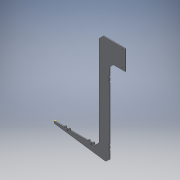
# Autodesk Inventor part: Z stage_side
Saved by Autodesk Inventor 2019 (Build 230136000, 136)
## iProperties
Created: 2020-03-07
Part Number: Z stage_side
Material: Generic
Document SubType Name: Modeling
Designer: Vijay
Density: 1 g/cm^3
Appearance: Default
Author: Vijay
Autodesk Inventor part; units mm, degrees
ref_plane "YZ Plane" through (0, 0, 0) normal (1, 0, 0) x (0, 1, 0)
ref_plane "XZ Plane" through (0, 0, 0) normal (0, 1, 0) x (-1, 0, 0)
ref_plane "XY Plane" through (0, 0, 0) normal (0, 0, 1) x (1, 0, 0)
sketch "Sketch1" plane through (0, 0, 0) normal (0, 0, 1) x (1, 0, 0)
  line L0 (230, 0) -> (0, 0) projected
  line L1 (0, 0) -> (0, -8.9243)
  line L2 (0, -8.9243) -> (282.1829, -48.5825)
  line L3 (282.1829, -48.5825) -> (282.1829, 400)
  line L4 (230, 0) -> (230, 500)
  line L5 (282.1829, 400) -> (362.1829, 400)
  line L6 (230, 500) -> (362.1829, 500)
  line L7 (362.1829, 500) -> (362.1829, 400)
  dimension "d0" = 400
  dimension "d1" = 8
  dimension "d10" = 80
  dimension "d11" = 100
  constraints: 14 end point, 2 horizontal, 2 vertical, 1 parallel, 1 perpendicular
  measures "d0" distance between parallel lines of L0 L5
  measures "d1" angle of L2 L0
  measures "d10" distance between parallel lines of L7 L3
  measures "d11" distance of L6.end L5.end
extrude "Extrusion1" add sketch "Sketch1" along normal blind 4
chamfer "Chamfer1" distance 20 angle 45 2 edges at (230, 500, 2) (282.1829, 400, 2)
chamfer "Chamfer2" distance 20 angle 45 2 edges at (230, 0, 2) (282.1829, -48.5825, 2)
sketch "Sketch2" plane through (0, 0, 0) normal (0, 0, -1) x (-1, 0, 0)
  point P0 (0, 0)
sketch "Sketch3" plane through (0, 0, 0) normal (0, 0, -1) x (-1, 0, 0)
  point P0 (0, 0)
sketch "Sketch4" plane through (0, 0, 0) normal (0, 0, -1) x (-1, 0, 0)
  point P0 (0, 0)
sketch "Sketch5" plane through (0, 0, 0) normal (0, 0, -1) x (-1, 0, 0)
  line L0 (-278.1829, 10.465) -> (-278.1829, 16.465) construction
  line L1 (-282.1829, 16.465) -> (-278.1829, 16.465) construction
  line L2 (-282.1829, 10.465) -> (-282.1829, 16.465) construction
  line L3 (-282.1829, 10.465) -> (-278.1829, 10.465) construction
  line L4 (-278.1829, 31.665) -> (-278.1829, 37.665) construction
  line L5 (-282.1829, 37.665) -> (-278.1829, 37.665) construction
  line L6 (-282.1829, 31.665) -> (-282.1829, 37.665) construction
  line L7 (-282.1829, 31.665) -> (-278.1829, 31.665) construction
  line L8 (-278.1829, 332.8339) -> (-278.1829, 338.8339) construction
  line L9 (-282.1829, 338.8339) -> (-278.1829, 338.8339) construction
  line L10 (-282.1829, 332.8339) -> (-282.1829, 338.8339) construction
  line L11 (-282.1829, 332.8339) -> (-278.1829, 332.8339) construction
  line L12 (-278.1829, 311.6339) -> (-278.1829, 317.6339) construction
  line L13 (-282.1829, 317.6339) -> (-278.1829, 317.6339) construction
  line L14 (-282.1829, 311.6339) -> (-282.1829, 317.6339) construction
  line L15 (-282.1829, 311.6339) -> (-278.1829, 311.6339) construction
  line L16 (-277.9829, 339.0339) -> (-277.9829, 332.6339)
  line L17 (-277.9829, 332.6339) -> (-282.3829, 332.6339)
  line L18 (-282.3829, 332.6339) -> (-282.3829, 339.0339)
  line L19 (-282.3829, 339.0339) -> (-277.9829, 339.0339)
  line L20 (-277.9829, 317.8339) -> (-277.9829, 311.4339)
  line L21 (-277.9829, 311.4339) -> (-282.3829, 311.4339)
  line L22 (-282.3829, 311.4339) -> (-282.3829, 317.8339)
  line L23 (-282.3829, 317.8339) -> (-277.9829, 317.8339)
  line L24 (-277.9829, 37.865) -> (-277.9829, 31.465)
  line L25 (-277.9829, 31.465) -> (-282.3829, 31.465)
  line L26 (-282.3829, 31.465) -> (-282.3829, 37.865)
  line L27 (-282.3829, 37.865) -> (-277.9829, 37.865)
  line L28 (-277.9829, 10.265) -> (-277.9829, 16.665)
  line L29 (-277.9829, 16.665) -> (-282.3829, 16.665)
  line L30 (-282.3829, 16.665) -> (-282.3829, 10.265)
  line L31 (-282.3829, 10.265) -> (-277.9829, 10.265)
  point P0 (0, 0)
  dimension "d24" = 0.2
  dimension "d25" = 0.2
  dimension "d26" = 0.2
  dimension "d27" = 0.2
  constraints: 32 end point, 12 other
  measures "d24" distance between parallel lines of L9 L19
  measures "d25" distance between parallel lines of L13 L23
  measures "d26" distance between parallel lines of L5 L27
  measures "d27" distance between parallel lines of L3 L31
extrude "Extrusion2" cut sketch "Sketch5" against normal blind 25.4
sketch "Sketch6" plane through (0, 0, 0) normal (0, 0, -1) x (-1, 0, 0)
  line L0 (-278.1829, 25.5649) -> (-278.1829, 22.5649) projected
  line L1 (-282.1829, 25.5649) -> (-278.1829, 25.5649) projected
  line L2 (-282.1829, 22.5649) -> (-282.1829, 25.5649) projected
  line L3 (-282.1829, 22.5649) -> (-278.1829, 22.5649) projected
  line L4 (-278.1829, 326.7338) -> (-278.1829, 323.7338) projected
  line L5 (-282.1829, 326.7338) -> (-278.1829, 326.7338) projected
  line L6 (-282.1829, 323.7338) -> (-282.1829, 326.7338) projected
  line L7 (-282.1829, 323.7338) -> (-278.1829, 323.7338) projected
  circle A0 centre (-280.1829, 325.2338) radius 1.6
  circle A1 centre (-280.1829, 24.0649) radius 1.6
  point P0 (0, 0)
  dimension "d14" = 3.2
  dimension "d15" = 3.2
  constraints: 2 centre point
  measures "d14" diameter of A0
  measures "d15" diameter of A1
extrude "Extrusion3" cut sketch "Sketch6" against normal through all contours A1 L3 L1 | L1 A1 | A1 L3 | A0 L7 L5 | L5 A0 | A0 L7
sketch "Sketch7" plane through (0, 0, 0) normal (0, 0, -1) x (-1, 0, 0)
  line L0 (-230, 4.0001) -> (-214.0001, 4.0001) projected
  line L1 (-210, 0) -> (-230, 20) projected
  line L2 (-210, 0) -> (-214.0001, 0)
  line L3 (-214.0001, 0) -> (-214.0001, 4.0001)
  line L4 (-214.0001, 4.0001) -> (-210, 4.0001)
  line L5 (-210, 4.0001) -> (-210, 0)
  point P0 (0, 0)
  constraints: 8 end point, 2 parallel, 2 point on line, 1 horizontal, 1 perpendicular
extrude "Extrusion4" cut sketch "Sketch7" against normal blind 25.4
sketch "Sketch8" plane through (0, 0, 0) normal (0, 0, -1) x (-1, 0, 0)
  line L0 (-209.8759, -14.6536) -> (-209.8759, 0) projected
  line L1 (-168.9242, -14.6536) -> (-209.8759, -14.6536) projected
  line L2 (-168.9242, 0) -> (-168.9242, -14.6536) projected
  line L3 (-175.8001, 0) -> (-168.9242, 0) projected
  line L4 (-175.8001, 6.35) -> (-175.8001, 0) projected
  line L5 (-181.8001, 6.35) -> (-175.8001, 6.35) projected
  line L6 (-181.8001, 0) -> (-181.8001, 6.35) projected
  line L7 (-187.9001, 0) -> (-181.8001, 0) projected
  line L8 (-187.9001, -6) -> (-187.9001, 0) projected
  line L9 (-186.6501, -6) -> (-187.9001, -6) projected
  line L10 (-186.6501, -8) -> (-186.6501, -6) projected
  line L11 (-187.9001, -8) -> (-186.6501, -8) projected
  line L12 (-187.9001, -10.65) -> (-187.9001, -8) projected
  line L13 (-190.9, -10.65) -> (-187.9001, -10.65) projected
  line L14 (-190.9, -8) -> (-190.9, -10.65) projected
  line L15 (-192.15, -8) -> (-190.9, -8) projected
  line L16 (-192.15, -6) -> (-192.15, -8) projected
  line L17 (-190.9, -6) -> (-192.15, -6) projected
  line L18 (-190.9, 0) -> (-190.9, -6) projected
  line L19 (-197, 0) -> (-190.9, 0) projected
  line L20 (-197, 6.35) -> (-197, 0) projected
  line L21 (-203.0001, 6.35) -> (-197, 6.35) projected
  line L22 (-203.0001, 0) -> (-203.0001, 6.35) projected
  line L23 (-209.8759, 0) -> (-203.0001, 0) projected
  line L24 (-88.9242, -14.6536) -> (-88.9242, 0) projected
  line L25 (-47.9725, -14.6536) -> (-88.9242, -14.6536) projected
  line L26 (-47.9725, 0) -> (-47.9725, -14.6536) projected
  line L27 (-54.8484, 0) -> (-47.9725, 0) projected
  line L28 (-54.8484, 6.35) -> (-54.8484, 0) projected
  line L29 (-60.8484, 6.35) -> (-54.8484, 6.35) projected
  line L30 (-60.8484, 0) -> (-60.8484, 6.35) projected
  line L31 (-66.9484, 0) -> (-60.8484, 0) projected
  line L32 (-66.9484, -6) -> (-66.9484, 0) projected
  line L33 (-65.6984, -6) -> (-66.9484, -6) projected
  line L34 (-65.6984, -8) -> (-65.6984, -6) projected
  line L35 (-66.9484, -8) -> (-65.6984, -8) projected
  line L36 (-66.9484, -10.65) -> (-66.9484, -8) projected
  line L37 (-69.9484, -10.65) -> (-66.9484, -10.65) projected
  line L38 (-69.9484, -8) -> (-69.9484, -10.65) projected
  line L39 (-71.1984, -8) -> (-69.9484, -8) projected
  line L40 (-71.1984, -6) -> (-71.1984, -8) projected
  line L41 (-69.9484, -6) -> (-71.1984, -6) projected
  line L42 (-69.9484, 0) -> (-69.9484, -6) projected
  line L43 (-76.0484, 0) -> (-69.9484, 0) projected
  line L44 (-76.0484, 6.35) -> (-76.0484, 0) projected
  line L45 (-82.0484, 6.35) -> (-76.0484, 6.35) projected
  line L46 (-82.0484, 0) -> (-82.0484, 6.35) projected
  line L47 (-88.9242, 0) -> (-82.0484, 0) projected
  point P0 (0, 0)
extrude "Extrusion5" add sketch "Sketch8" against normal up to surface (4 mm away)
sketch "Sketch10" plane through (0, 0, 0) normal (0, 0, -1) x (-1, 0, 0)
  line L0 (-209.8759, -14.6536) -> (-209.8759, 0) projected
  line L1 (-168.9242, -14.6536) -> (-209.8759, -14.6536) projected
  line L2 (-168.9242, 0) -> (-168.9242, -14.6536) projected
  line L3 (-175.8001, 0) -> (-168.9242, 0) projected
  line L4 (-175.8001, 6.35) -> (-175.8001, 0) projected
  line L5 (-181.8001, 6.35) -> (-175.8001, 6.35) projected
  line L6 (-181.8001, 0) -> (-181.8001, 6.35) projected
  line L7 (-187.9001, 0) -> (-181.8001, 0) projected
  line L8 (-187.9001, -6) -> (-187.9001, 0) projected
  line L9 (-186.6501, -6) -> (-187.9001, -6) projected
  line L10 (-186.6501, -8) -> (-186.6501, -6) projected
  line L11 (-187.9001, -8) -> (-186.6501, -8) projected
  line L12 (-187.9001, -10.65) -> (-187.9001, -8) projected
  line L13 (-190.9, -10.65) -> (-187.9001, -10.65) projected
  line L14 (-190.9, -8) -> (-190.9, -10.65) projected
  line L15 (-192.15, -8) -> (-190.9, -8) projected
  line L16 (-192.15, -6) -> (-192.15, -8) projected
  line L17 (-190.9, -6) -> (-192.15, -6) projected
  line L18 (-190.9, 0) -> (-190.9, -6) projected
  line L19 (-197, 0) -> (-190.9, 0) projected
  line L20 (-197, 6.35) -> (-197, 0) projected
  line L21 (-203.0001, 6.35) -> (-197, 6.35) projected
  line L22 (-203.0001, 0) -> (-203.0001, 6.35) projected
  line L23 (-209.8759, 0) -> (-203.0001, 0) projected
  line L24 (-88.9242, -14.6536) -> (-88.9242, 0) projected
  line L25 (-47.9725, -14.6536) -> (-88.9242, -14.6536) projected
  line L26 (-47.9725, 0) -> (-47.9725, -14.6536) projected
  line L27 (-54.8484, 0) -> (-47.9725, 0) projected
  line L28 (-54.8484, 6.35) -> (-54.8484, 0) projected
  line L29 (-60.8484, 6.35) -> (-54.8484, 6.35) projected
  line L30 (-60.8484, 0) -> (-60.8484, 6.35) projected
  line L31 (-66.9484, 0) -> (-60.8484, 0) projected
  line L32 (-66.9484, -6) -> (-66.9484, 0) projected
  line L33 (-65.6984, -6) -> (-66.9484, -6) projected
  line L34 (-65.6984, -8) -> (-65.6984, -6) projected
  line L35 (-66.9484, -8) -> (-65.6984, -8) projected
  line L36 (-66.9484, -10.65) -> (-66.9484, -8) projected
  line L37 (-69.9484, -10.65) -> (-66.9484, -10.65) projected
  line L38 (-69.9484, -8) -> (-69.9484, -10.65) projected
  line L39 (-71.1984, -8) -> (-69.9484, -8) projected
  line L40 (-71.1984, -6) -> (-71.1984, -8) projected
  line L41 (-69.9484, -6) -> (-71.1984, -6) projected
  line L42 (-69.9484, 0) -> (-69.9484, -6) projected
  line L43 (-76.0484, 0) -> (-69.9484, 0) projected
  line L44 (-76.0484, 6.35) -> (-76.0484, 0) projected
  line L45 (-82.0484, 6.35) -> (-76.0484, 6.35) projected
  line L46 (-82.0484, 0) -> (-82.0484, 6.35) projected
  line L47 (-88.9242, 0) -> (-82.0484, 0) projected
  line L48 (-190.9, 0) -> (-187.9001, 0)
  line L49 (-197, 0) -> (-181.8001, 0) projected
  line L50 (-69.9484, 0) -> (-66.9484, 0)
  line L51 (-76.0484, 0) -> (-60.8484, 0) projected
  point P0 (0, 0)
  constraints: 4 end point, 2 collinear
extrude "Extrusion6" cut sketch "Sketch10" against normal blind 25.4 contours L48 L8 L9 L10 L11 L12 L13 L14 L15 L16 L17 L18 | L50 L32 L33 L34 L35 L36 L37 L38 L39 L40 L41 L42
sketch "Sketch11" plane through (0, 0, 0) normal (0, 0, -1) x (-1, 0, 0)
  line L0 (-342.1829, 500) -> (-342.1829, 400) projected
  circle A0 centre (-352.1829, 490) radius 3
  circle A1 centre (-352.1829, 410) radius 3
  line L1 (-362.1829, 500) -> (-362.1829, 400) projected
  line L2 (-250, 500) -> (-362.1829, 500) projected
  line L3 (-362.1829, 400) -> (-302.1829, 400) projected
  point P0 (0, 0)
  dimension "d28" = 6
  dimension "d29" = 6
  dimension "d30" = 10
  dimension "d31" = 10
  dimension "d32" = 10
  dimension "d33" = 10
  constraints: 2 centre point
  measures "d28" diameter of A0
  measures "d29" diameter of A1
  measures "d30" distance from line of L1 A0.centre
  measures "d31" distance from line of L1 A1.centre
  measures "d32" distance from line of L2 A0.centre
  measures "d33" distance from line of L3 A1.centre
extrude "Extrusion7" cut sketch "Sketch11" against normal blind 25.4 contours A0 | A1
sketch "Sketch12" plane through (0, 0, 4) normal (0, 0, 1) x (1, 0, 0)
  circle A0 centre (352.1829, 490) radius 3 projected
  circle A1 centre (352.1829, 410) radius 3 projected
  line L0 (187.9001, -6) -> (187.9001, 0) projected
  line L1 (187.9001, 0) -> (181.8001, 0) projected
  line L2 (181.8001, 6.35) -> (181.8001, 0) projected
  line L3 (175.8001, 6.35) -> (181.8001, 6.35) projected
  line L4 (175.8001, 0) -> (175.8001, 6.35) projected
  line L5 (175.8001, 0) -> (82.0484, 0) projected
  line L6 (82.0484, 6.35) -> (82.0484, 0) projected
  line L7 (76.0484, 6.35) -> (82.0484, 6.35) projected
  line L8 (76.0484, 0) -> (76.0484, 6.35) projected
  line L9 (76.0484, 0) -> (69.9484, 0) projected
  line L10 (69.9484, 0) -> (69.9484, -6) projected
  line L11 (69.9484, -6) -> (71.1984, -6) projected
  line L12 (71.1984, -6) -> (71.1984, -8) projected
  line L13 (71.1984, -8) -> (69.9484, -8) projected
  line L14 (69.9484, -8) -> (69.9484, -10.65) projected
  line L15 (69.9484, -10.65) -> (66.9484, -10.65) projected
  line L16 (66.9484, -10.65) -> (66.9484, -8) projected
  line L17 (66.9484, -8) -> (65.6984, -8) projected
  line L18 (65.6984, -8) -> (65.6984, -6) projected
  line L19 (65.6984, -6) -> (66.9484, -6) projected
  line L20 (66.9484, -6) -> (66.9484, 0) projected
  line L21 (66.9484, 0) -> (60.8484, 0) projected
  line L22 (60.8484, 6.35) -> (60.8484, 0) projected
  line L23 (54.8484, 6.35) -> (60.8484, 6.35) projected
  line L24 (54.8484, 0) -> (54.8484, 6.35) projected
  line L25 (54.8484, 0) -> (0, 0) projected
  line L26 (0, 0) -> (0, -8.9243) projected
  line L27 (0, -8.9243) -> (262.3776, -45.7991) projected
  line L28 (282.1829, -28.5825) -> (262.3776, -45.7991) projected
  line L29 (282.1829, -28.5825) -> (282.1829, 10.265) projected
  line L30 (282.1829, 10.265) -> (277.9829, 10.265) projected
  line L31 (277.9829, 10.265) -> (277.9829, 16.665) projected
  line L32 (277.9829, 16.665) -> (282.1829, 16.665) projected
  line L33 (282.1829, 16.665) -> (282.1829, 31.465) projected
  line L34 (282.1829, 31.465) -> (277.9829, 31.465) projected
  line L35 (277.9829, 31.465) -> (277.9829, 37.865) projected
  line L36 (277.9829, 37.865) -> (282.1829, 37.865) projected
  line L37 (282.1829, 37.865) -> (282.1829, 311.4339) projected
  line L38 (282.1829, 311.4339) -> (277.9829, 311.4339) projected
  line L39 (277.9829, 311.4339) -> (277.9829, 317.8339) projected
  line L40 (277.9829, 317.8339) -> (282.1829, 317.8339) projected
  line L41 (282.1829, 317.8339) -> (282.1829, 332.6339) projected
  line L42 (282.1829, 332.6339) -> (277.9829, 332.6339) projected
  line L43 (277.9829, 332.6339) -> (277.9829, 339.0339) projected
  line L44 (277.9829, 339.0339) -> (282.1829, 339.0339) projected
  line L45 (282.1829, 339.0339) -> (282.1829, 380) projected
  line L46 (302.1829, 400) -> (282.1829, 380) projected
  line L47 (302.1829, 400) -> (362.1829, 400) projected
  line L48 (362.1829, 400) -> (362.1829, 500) projected
  line L49 (362.1829, 500) -> (250, 500) projected
  line L50 (230, 480) -> (250, 500) projected
  line L51 (230, 480) -> (230, 20) projected
  line L52 (214.0001, 4.0001) -> (230, 20) projected
  line L53 (214.0001, 4.0001) -> (214.0001, 0) projected
  line L54 (214.0001, 0) -> (203.0001, 0) projected
  line L55 (203.0001, 6.35) -> (203.0001, 0) projected
  line L56 (197, 6.35) -> (203.0001, 6.35) projected
  line L57 (197, 0) -> (197, 6.35) projected
  line L58 (197, 0) -> (190.9, 0) projected
  line L59 (190.9, 0) -> (190.9, -6) projected
  line L60 (190.9, -6) -> (192.15, -6) projected
  line L61 (192.15, -6) -> (192.15, -8) projected
  line L62 (192.15, -8) -> (190.9, -8) projected
  line L63 (190.9, -8) -> (190.9, -10.65) projected
  line L64 (190.9, -10.65) -> (187.9001, -10.65) projected
  line L65 (187.9001, -10.65) -> (187.9001, -8) projected
  line L66 (187.9001, -8) -> (186.6501, -8) projected
  line L67 (186.6501, -8) -> (186.6501, -6) projected
  line L68 (186.6501, -6) -> (187.9001, -6) projected
  circle A2 centre (280.1829, 24.0649) radius 1.6 projected
  circle A3 centre (280.1829, 325.2338) radius 1.6 projected
  line L69 (66.7484, -0.2) -> (66.7484, -5.8)
  line L70 (66.7484, -5.8) -> (65.4984, -5.8)
  line L71 (65.4984, -5.8) -> (65.4984, -8.2)
  line L72 (65.4984, -8.2) -> (66.7484, -8.2)
  line L73 (66.7484, -8.2) -> (66.7484, -10.85)
  line L74 (66.7484, -10.85) -> (70.1484, -10.85)
  line L75 (70.1484, -10.85) -> (70.1484, -8.2)
  line L76 (70.1484, -8.2) -> (71.3984, -8.2)
  line L77 (71.3984, -8.2) -> (71.3984, -5.8)
  line L78 (71.3984, -5.8) -> (70.1484, -5.8)
  line L79 (70.1484, -5.8) -> (70.1484, -0.2)
  line L80 (76.2484, -0.2) -> (76.2484, 6.15)
  line L81 (76.2484, 6.15) -> (81.8484, 6.15)
  line L82 (81.8484, 6.15) -> (81.8484, -0.2)
  line L83 (81.8484, -0.2) -> (176.0001, -0.2)
  line L84 (176.0001, -0.2) -> (176.0001, 6.15)
  line L85 (176.0001, 6.15) -> (181.6001, 6.15)
  line L86 (181.6001, 6.15) -> (181.6001, -0.2)
  line L87 (187.7001, -0.2) -> (187.7001, -5.8)
  line L88 (187.7001, -5.8) -> (186.4501, -5.8)
  line L89 (186.4501, -5.8) -> (186.4501, -8.2)
  line L90 (186.4501, -8.2) -> (187.7001, -8.2)
  line L91 (187.7001, -8.2) -> (187.7001, -10.85)
  line L92 (187.7001, -10.85) -> (191.1, -10.85)
  line L93 (191.1, -10.85) -> (191.1, -8.2)
  line L94 (191.1, -8.2) -> (192.35, -8.2)
  line L95 (192.35, -8.2) -> (192.35, -5.8)
  line L96 (192.35, -5.8) -> (191.1, -5.8)
  line L97 (191.1, -5.8) -> (191.1, -0.2)
  line L98 (197.2, -0.2) -> (197.2, 6.15)
  line L99 (197.2, 6.15) -> (202.8001, 6.15)
  line L100 (202.8001, 6.15) -> (202.8001, -0.2)
  line L101 (202.8001, -0.2) -> (214.2001, -0.2)
  line L102 (214.2001, -0.2) -> (214.2001, 3.9172)
  line L103 (214.2001, 3.9172) -> (230.2, 19.9172)
  line L104 (230.2, 19.9172) -> (230.2, 479.9172)
  line L105 (230.2, 479.9172) -> (250.0828, 499.8)
  line L106 (250.0828, 499.8) -> (361.9829, 499.8)
  line L107 (361.9829, 499.8) -> (361.9829, 400.2)
  line L108 (361.9829, 400.2) -> (302.1001, 400.2)
  line L109 (302.1001, 400.2) -> (281.9829, 380.0828)
  line L110 (281.9829, 380.0828) -> (281.9829, 339.2339)
  line L111 (281.9829, 339.2339) -> (277.7829, 339.2339)
  line L112 (277.7829, 339.2339) -> (277.7829, 332.4339)
  line L113 (277.7829, 332.4339) -> (281.9829, 332.4339)
  line L114 (281.9829, 332.4339) -> (281.9829, 318.0339)
  line L115 (281.9829, 318.0339) -> (277.7829, 318.0339)
  line L116 (277.7829, 318.0339) -> (277.7829, 311.2339)
  line L117 (277.7829, 311.2339) -> (281.9829, 311.2339)
  line L118 (281.9829, 311.2339) -> (281.9829, 38.065)
  line L119 (281.9829, 38.065) -> (277.7829, 38.065)
  line L120 (277.7829, 38.065) -> (277.7829, 31.265)
  line L121 (277.7829, 31.265) -> (281.9829, 31.265)
  line L122 (281.9829, 31.265) -> (281.9829, 16.865)
  line L123 (281.9829, 16.865) -> (277.7829, 16.865)
  line L124 (277.7829, 16.865) -> (277.7829, 10.065)
  line L125 (277.7829, 10.065) -> (281.9829, 10.065)
  line L126 (281.9829, 10.065) -> (281.9829, -28.4914)
  line L127 (281.9829, -28.4914) -> (262.3152, -45.5883)
  line L128 (262.3152, -45.5883) -> (0.2, -8.7504)
  line L129 (0.2, -8.7504) -> (0.2, -0.2)
  line L130 (0.2, -0.2) -> (55.0484, -0.2)
  line L131 (55.0484, -0.2) -> (55.0484, 6.15)
  line L132 (55.0484, 6.15) -> (60.6484, 6.15)
  line L133 (60.6484, 6.15) -> (60.6484, -0.2)
  line L134 (69.9484, 0) -> (76.0484, 0) projected
  line L135 (70.1484, -0.2) -> (70.1484, 0)
  line L136 (70.1484, 0) -> (66.7484, 0)
  line L137 (66.7484, 0) -> (66.7484, -0.2)
  line L138 (190.9, 0) -> (197, 0) projected
  line L139 (191.1, -0.2) -> (191.1, 0)
  line L140 (191.1, 0) -> (187.7001, 0)
  line L141 (187.7001, 0) -> (187.7001, -0.2)
  line L142 (181.6001, -0.2) -> (181.8001, -0.2)
  line L143 (197, -0.2) -> (197.2, -0.2)
  dimension "d36" = 0.2
  constraints: 146 end point, 4 point on line, 2 parallel, 61 other
  measures "d36" distance between parallel lines of L20 L69
extrude "Extrusion8" cut sketch "Sketch12" against normal blind 25.4 contours L68 L67 L66 L65 L64 L63 L62 L61 L60 L59 L58 L139 L97 L96 L95 L94 L93 L92 L91 L90 L89 L88 L87 L141 L1 L0 | L0 L140 L59 L60 L61 L62 L63 L64 L65 L66 L67 L68 | L135 L79 L78 L77 L76 L75 L74 L73 L72 L71 L70 L69 L137 L21 L20 L19 L18 L17 L16 L15 L14 L13 L12 L11 L10 L9 | L10 L11 L12 L13 L14 L15 L16 L17 L18 L19 L20 L136
body "Solid1"
